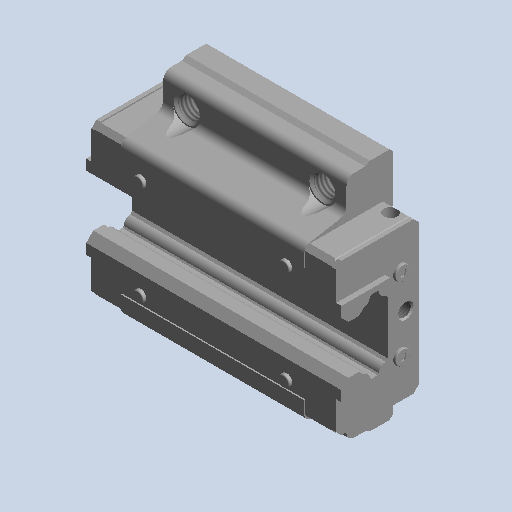
# Autodesk Inventor part: HSR30ASSB-M6F1 Slider-1
Saved by Autodesk Inventor 2022 (Build 260153000, 153)
## iProperties
Part Number: HSR30ASSB-M6F1 Slider-1
Material: Generic
Catalog Web Link: www.cadenas.de
Description: Flange Type - Heavy Load HSR-A Slider-Slider
Vendor: THK
Document SubType Name: Modeling
Designer: partserver
Manufacturer: THK
Mass: 181.354 g
Surface Area: 319.293 cm^2
Volume: 181.354 cm^3
Density: 1 g/cm^3
Appearance: PSOLRGB-192-192-192
Category: PARTsolutions
Company: THK
PSOL_IDENT_0: {$CADENAS_DATA\23d-libs\thk\linear_motion_systems\lm_guide\lm_guide\lm_guide_hsr\four_taped_hole_typ
PSOL_IDENT_1: e\hsr_a\hsr_a_slider.prj},234 {VTYP=3D},{NB=HSR30ASSB-M6F1 Slider-1},{LINA=HSR30ASSB-M6F1 Slider-1},
PSOL_IDENT_2: {NN=Flange Type - Heavy Load HSR-A Slider},{DATE=08.06.2021 00:57:44},{GEOMDATE=03.12.2020 11:07:00}
PSOL_IDENT_3: ,{VERSION=},{LINEID=70},{WBVAR=SO,QZ,GPJ,TH,XY},{WBNUMERIC=XY}  {NB=HSR30ASSB-M6F1 Slider-1},{LINA=H
PSOL_IDENT_4: SR30ASSB-M6F1 Slider-1},{KT=DUMMY},{MN=HSR30A},{SO=SS},{QZ=},{GPJ=B-M6F},{TH=1},{SO1='SS','SS- With
PSOL_IDENT_5: end, side seals','','Without Seals','UU','UU- With end seals (on both ends)','DD','DD- With double,
PSOL_IDENT_6: side, inner seals','ZZ','ZZ- With end, side, inner seals and metal scrapers','KK','KK- With double,
PSOL_IDENT_7: side, inner seals and metal scrapers','SSHH','SSHH- With end, side, inner seals and LaCS','DDHH','DD
PSOL_IDENT_8: HH- With double, side, inner seals and LaCS','ZZHH','ZZHH- With end, side, inner seals and metal scr
PSOL_IDENT_9: apers and LaCS','KKHH','KKHH- With double, side, inner seals and metal scrapers and LaCS'},{M=42.00}
PSOL_IDENT_10: ,{W=90.00},{L=98.00},{B=72.00},{C=52.00},{S=10.00},{L1=70.40},{SST=0.000},{T=9.000},{T1=18.000},{K=3
PSOL_IDENT_11: 5.00},{N=7.00},{H3=7.000},{W1=28.000},{M1=26.000},{LX=98},{LL1=0.000},{SH=58.00},{Z1=2.000},{Z2=2.00
PSOL_IDENT_12: 0},{GPJ1=<'B-M6F','B-M6F'>,'', 'None', 'A-M6F','A-M6F','C-M6F','C-M6F', 'LF-A','LF-A','LF-B','LF-B',
PSOL_IDENT_13: 'SF-A','SF-A','SF-B','SF-B'},{L4=0.95},{ND=4.000},{SE=58.000},{SE3=2.000},{SE4=2.000},{V=38.000},{V
PSOL_IDENT_14: 1=56.000},{V2=4.370},{V3=1.283},{ST=31.717},{SE1=31.717},{SU=1.283},{SE2=1.283},{STT=2.000},{SEE1=2.
PSOL_IDENT_15: 000},{UP=1.283},{QZX='','No','QZ','Yes'},{LP=2},{L3=10.300},{L5=2},{S2=5.500},{L7=0.000},{XX=28.000}
PSOL_IDENT_16: ,{R=2.850},{YY=26.000},{SS=2.500},{ZZ=0.000},{GPJX=2},{X=2},{E0=5.200},{F0=6.200},{D0=5.200},{D2=6.2
PSOL_IDENT_17: 00},{E1=5.200},{SD2=1.00},{XY=1},{WX=11.000},{H1=1.000},{H2=0.400},{RX=19.500},{D=6.200},{LL=5.120},
PSOL_IDENT_18: {TX=1.000},{NOTE=MIN}
NB: HSR30ASSB-M6F1 Slider-1
NN: Flange Type - Heavy Load HSR-A Slider
NT: Slider
NBSYN: $MN.$SO.$QZ.$GPJ.$TH. Slider-$XY.
LINA: HSR30ASSB-M6F1 Slider-1
CATALOG: THK
MN: HSR30A
SO: SS- With end, side seals
QZ: No
GPJ: B-M6F
TH: on
M: 42
W: 90
L: 98
B: 72
C: 52
S: 10
L1: 70.4
SST: 0
T: 9
T1: 18
K: 35
N: 7
H3: 7
W1: 28
M1: 26
LL1: 0
SH: 58
Z1: 2
Z2: 2
ND: 4
SE: 58
SE3: 2
SE4: 2
V: 38
V1: 56
V2: 4.37
V3: 1.283
SU: 1.283
SE2: 1.283
STT: 2
SEE1: 2
L3: 10.3
S2: 5.5
L7: 0
XX: 28
R: 2.85
YY: 26
SS: 2.5
ZZ: 0
E0: 5.2
F0: 6.2
D0: 5.2
D2: 6.2
E1: 5.2
SD2: 1
XY: 1
WX: 11
H1: 1
H2: 0.4
RX: 19.5
D: 6.2
LL: 5.12
TX: 1
NOTE: 0
SUPPLIER: THK
ARTICLENO: HSR30ASSB-M6F1 Slider-1
BOMINFO: HSR30ASSB-M6F1 Slider-1
CREATOR: CADENAS GmbH
Title: HSR30ASSB-M6F1 Slider-1
Author: Cadenas PARTsolutions
Comments: Slider
Autodesk Inventor part; units mm, degrees
sketch "Sketch_17" plane through (0, 0, 0) normal (1, 0, 0) x (0, 1, 0)
  line L0 (33.6, 45) -> (26, 45)
  line L1 (26, 45) -> (24.268, 44)
  line L2 (24.268, 44) -> (20, 44)
  arc A0 (20, 44) -> (17, 41) centre (20, 41) ccw
  line L3 (17, 41) -> (17, 34.3433)
  arc A1 (14.514, 31.3877) -> (17, 34.3433) centre (14, 34.3433) ccw
  line L4 (14.514, 31.3877) -> (3.269, 29.4323)
  arc A2 (3.269, 29.4323) -> (0.783, 26.4767) centre (3.783, 26.4767) ccw
  line L5 (0.783, 26.4767) -> (0.783, 22)
  line L6 (0.783, 22) -> (1.283, 22)
  line L7 (1.283, 22) -> (1.283, -22)
  line L8 (1.283, -22) -> (0.783, -22)
  line L9 (0.783, -22) -> (0.783, -26.4767)
  arc A3 (0.783, -26.4767) -> (3.269, -29.4323) centre (3.783, -26.4767) ccw
  line L10 (3.269, -29.4323) -> (14.514, -31.3877)
  arc A4 (17, -34.3433) -> (14.514, -31.3877) centre (14, -34.3433) ccw
  line L11 (17, -34.3433) -> (17, -41)
  arc A5 (17, -41) -> (20, -44) centre (20, -41) ccw
  line L12 (20, -44) -> (24.268, -44)
  line L13 (24.268, -44) -> (26, -45)
  line L14 (26, -45) -> (33.6, -45)
  line L15 (33.6, -45) -> (35, -43.6)
  line L16 (35, -43.6) -> (35, -25.8)
  line L17 (35, -25.8) -> (34.2, -25)
  line L18 (34.2, -25) -> (34.2, -11)
  line L19 (34.2, -11) -> (35, -10.2)
  line L20 (35, -10.2) -> (35, 10.2)
  line L21 (35, 10.2) -> (34.2, 11)
  line L22 (34.2, 11) -> (34.2, 25)
  line L23 (34.2, 25) -> (35, 25.8)
  line L24 (35, 25.8) -> (35, 43.6)
  line L25 (35, 43.6) -> (33.6, 45)
  constraints: 52 end point, 12 point on circle, 6 centre point
extrude "Extrusion1" add sketch "Sketch_17" along normal mid plane 70.4
sketch "Sketch_28" plane through (0, 0, 36) normal (0, 0, 1) x (1, 0, 0)
  line L0 (-26, 35) -> (-26, 17)
  line L1 (-26, 17) -> (-31, 17)
  line L2 (-31, 17) -> (-30.188, 17.812)
  line L3 (-30.188, 17.812) -> (-30.188, 34.188)
  line L4 (-30.188, 34.188) -> (-31, 35)
  line L5 (-31, 35) -> (-26, 35)
  line L6 (-26, 35) -> (-26, 17)
  constraints: 14 end point
revolve "Revolution1" cut sketch "Sketch_28" angle 360 about axis through (-26, 35, 36) along (0, 1, 0)
thread "Thread1" size "M10x1.5" class "6H" standard "ISO Metric profile" full length
pattern_linear "Rectangular Pattern1" count 2 spacing 52 along (1, 0, 0) count 2 spacing 72 along (0, 0, -1) of "Revolution1"
sketch "Sketch_60" plane through (0, 17, 0) normal (0, 1, 0) x (1, 0, 0)
  line L0 (-31.5, -36) -> (-31.5, -53.5)
  line L1 (-31.5, -53.5) -> (-20.5, -53.5)
  line L2 (-20.5, -53.5) -> (-20.5, -36)
  arc A0 (-20.5, -36) -> (-31.5, -36) centre (-26, -36) ccw
  constraints: 6 end point, 2 point on circle, 1 centre point
extrude "Extrusion2" cut sketch "Sketch_60" against normal blind 35
sketch "Sketch_61" plane through (0, 17, 0) normal (0, 1, 0) x (1, 0, 0)
  arc A0 (-31.5, 36) -> (-20.5, 36) centre (-26, 36) ccw
  line L0 (-20.5, 36) -> (-20.5, 53.5)
  line L1 (-20.5, 53.5) -> (-31.5, 53.5)
  line L2 (-31.5, 53.5) -> (-31.5, 36)
  constraints: 6 end point, 2 point on circle, 1 centre point
extrude "Extrusion3" cut sketch "Sketch_61" against normal blind 17
sketch "Sketch_62" plane through (0, 17, 0) normal (0, 1, 0) x (1, 0, 0)
  line L0 (20.5, -36) -> (20.5, -53.5)
  line L1 (20.5, -53.5) -> (31.5, -53.5)
  line L2 (31.5, -53.5) -> (31.5, -36)
  arc A0 (31.5, -36) -> (20.5, -36) centre (26, -36) ccw
  constraints: 6 end point, 2 point on circle, 1 centre point
extrude "Extrusion4" cut sketch "Sketch_62" against normal blind 17
sketch "Sketch_63" plane through (0, 17, 0) normal (0, 1, 0) x (1, 0, 0)
  arc A0 (20.5, 36) -> (31.5, 36) centre (26, 36) ccw
  line L0 (31.5, 36) -> (31.5, 53.5)
  line L1 (31.5, 53.5) -> (20.5, 53.5)
  line L2 (20.5, 53.5) -> (20.5, 36)
  constraints: 6 end point, 2 point on circle, 1 centre point
extrude "Extrusion5" cut sketch "Sketch_63" against normal blind 17
sketch "Sketch_7" plane through (-45.5, 0, 0) normal (1, 0, 0) x (0, 0, -1)
  line L0 (-29, 2.983) -> (-27.3, 1.283)
  line L1 (-27.3, 1.283) -> (27.3, 1.283)
  line L2 (27.3, 1.283) -> (29, 2.983)
  line L3 (29, 2.983) -> (29, 31)
  line L4 (29, 31) -> (27, 33)
  line L5 (27, 33) -> (-27, 33)
  line L6 (-27, 33) -> (-29, 31)
  line L7 (-29, 31) -> (-29, 2.983)
  constraints: 16 end point
extrude "Extrusion6" add sketch "Sketch_7" along normal blind 10.3
sketch "Sketch_2" plane through (-45.5, 0, 0) normal (1, 0, 0) x (0, 0, -1)
  line L0 (-29, 3.283) -> (-27, 1.283)
  line L1 (-27, 1.283) -> (27, 1.283)
  line L2 (27, 1.283) -> (29, 3.283)
  line L3 (29, 3.283) -> (29, 31)
  line L4 (29, 31) -> (27, 33)
  line L5 (27, 33) -> (-27, 33)
  line L6 (-27, 33) -> (-29, 31)
  line L7 (-29, 31) -> (-29, 3.283)
  constraints: 16 end point
extrude "Extrusion7" add sketch "Sketch_2" against normal blind 3.5
sketch "Sketch_8" plane through (45.5, 0, 0) normal (1, 0, 0) x (0, 0, -1)
  line L0 (-29, 2.983) -> (-27.3, 1.283)
  line L1 (-27.3, 1.283) -> (27.3, 1.283)
  line L2 (27.3, 1.283) -> (29, 2.983)
  line L3 (29, 2.983) -> (29, 31)
  line L4 (29, 31) -> (27, 33)
  line L5 (27, 33) -> (-27, 33)
  line L6 (-27, 33) -> (-29, 31)
  line L7 (-29, 31) -> (-29, 2.983)
  constraints: 16 end point
extrude "Extrusion8" add sketch "Sketch_8" against normal blind 10.3
sketch "Sketch_107" plane through (-35.2, 0, 0) normal (1, 0, 0) x (0, 0, -1)
  line L0 (-10.3, 32.5) -> (10.3, 32.5)
  line L1 (10.3, 32.5) -> (10.3, 34)
  arc A0 (5.5, 34.6) -> (10.3, 34) centre (10.3, 53.5) ccw
  line L2 (5.5, 34.6) -> (-5.5, 34.6)
  arc A1 (-10.3, 34) -> (-5.5, 34.6) centre (-10.3, 53.5) ccw
  line L3 (-10.3, 34) -> (-10.3, 32.5)
  constraints: 8 end point, 4 point on circle, 2 centre point
extrude "Extrusion9" add sketch "Sketch_107" against normal blind 9.8
sketch "Sketch_9" plane through (45.5, 0, 0) normal (1, 0, 0) x (0, 0, -1)
  line L0 (-29, 3.283) -> (-27, 1.283)
  line L1 (-27, 1.283) -> (27, 1.283)
  line L2 (27, 1.283) -> (29, 3.283)
  line L3 (29, 3.283) -> (29, 31)
  line L4 (29, 31) -> (27, 33)
  line L5 (27, 33) -> (-27, 33)
  line L6 (-27, 33) -> (-29, 31)
  line L7 (-29, 31) -> (-29, 3.283)
  constraints: 16 end point
extrude "Extrusion10" add sketch "Sketch_9" along normal blind 3.5
sketch "Sketch_106" plane through (35.2, 0, 0) normal (1, 0, 0) x (0, 0, -1)
  line L0 (-10.3, 32.5) -> (10.3, 32.5)
  line L1 (10.3, 32.5) -> (10.3, 34)
  arc A0 (5.5, 34.6) -> (10.3, 34) centre (10.3, 53.5) ccw
  line L2 (5.5, 34.6) -> (-5.5, 34.6)
  arc A1 (-10.3, 34) -> (-5.5, 34.6) centre (-10.3, 53.5) ccw
  line L3 (-10.3, 34) -> (-10.3, 32.5)
  constraints: 8 end point, 4 point on circle, 2 centre point
extrude "Extrusion11" add sketch "Sketch_106" along normal blind 9.8
sketch "Sketch13" plane through (-45, 34.6, -5.5) normal (0, 1, 0) x (1, 0, 0)
  point P0 (4.68, -5.5)
hole "Hole1" at (-40.32, 34.6, 0) direction (0, -1, 0) diameter 6.2 depth 1
sketch "Sketch14" plane through (35.2, 34.6, 5.5) normal (0, 1, 0) x (1, 0, 0)
  point P0 (5.12, 5.5)
hole "Hole2" at (40.32, 34.6, 0) direction (0, -1, 0) diameter 6.2 depth 1
sketch "Sketch_1" plane through (49, 0, 0) normal (1, 0, 0) x (0, 0, -1)
  line L0 (-29, 35) -> (-29, 0)
  line L1 (-29, 0) -> (29, 0)
  line L2 (29, 0) -> (29, 35)
  line L3 (29, 35) -> (-29, 35)
  constraints: 8 end point
extrude "Extrusion12" cut sketch "Sketch_1" against normal blind 2
sketch "Sketch_6" plane through (-49, 0, 0) normal (1, 0, 0) x (0, 0, -1)
  line L0 (-29, 35) -> (-29, 0)
  line L1 (-29, 0) -> (29, 0)
  line L2 (29, 0) -> (29, 35)
  line L3 (29, 35) -> (-29, 35)
  constraints: 8 end point
extrude "Extrusion13" cut sketch "Sketch_6" along normal blind 2
sketch "Sketch_20" plane through (-47, 0, 0) normal (1, 0, 0) x (0, 0, -1)
  line L0 (-16, 1.283) -> (16, 1.283)
  line L1 (16, 1.283) -> (16, 20)
  line L2 (16, 20) -> (15, 21)
  line L3 (15, 21) -> (-15, 21)
  line L4 (-15, 21) -> (-16, 20)
  line L5 (-16, 20) -> (-16, 1.283)
  constraints: 12 end point
extrude "Extrusion14" add sketch "Sketch_20" against normal blind 2
sketch "Sketch_21" plane through (47, 0, 0) normal (1, 0, 0) x (0, 0, -1)
  line L0 (-16, 1.283) -> (16, 1.283)
  line L1 (16, 1.283) -> (16, 20)
  line L2 (16, 20) -> (15, 21)
  line L3 (15, 21) -> (-15, 21)
  line L4 (-15, 21) -> (-16, 20)
  line L5 (-16, 20) -> (-16, 1.283)
  constraints: 12 end point
extrude "Extrusion15" add sketch "Sketch_21" along normal blind 2
sketch "Sketch_64" plane through (0, 0, 0) normal (1, 0, 0) x (0, 1, 0)
  line L0 (-5.5, 14) -> (-7, 12.5)
  line L1 (-7, 12.5) -> (-7, 7.75)
  line L2 (-7, 7.75) -> (-6.5, 7.25)
  line L3 (-6.5, 7.25) -> (-6.5, 3.75)
  line L4 (-6.5, 3.75) -> (-7, 3.25)
  line L5 (-7, 3.25) -> (-7, -3.25)
  line L6 (-7, -3.25) -> (-6.5, -3.75)
  line L7 (-6.5, -3.75) -> (-6.5, -7.25)
  line L8 (-6.5, -7.25) -> (-7, -7.75)
  line L9 (-7, -7.75) -> (-7, -12.5)
  line L10 (-7, -12.5) -> (-5.5, -14)
  line L11 (-5.5, -14) -> (-0.7, -14)
  line L12 (-0.7, -14) -> (3.9996, -9.3003)
  line L13 (3.9996, -9.3003) -> (8.0794, -9.3003)
  line L14 (8.0794, -9.3003) -> (9.7787, -10.9996)
  arc A0 (12.31, -13.5309) -> (9.7787, -10.9996) centre (9.4399, -13.8696) ccw
  line L15 (12.31, -13.5309) -> (12.7791, -14)
  line L16 (12.7791, -14) -> (15.215, -14)
  line L17 (15.215, -14) -> (15.6905, -13.5245)
  arc A1 (18.2147, -11.0003) -> (15.6905, -13.5245) centre (18.5598, -13.8696) ccw
  line L18 (18.2147, -11.0003) -> (19, -10.215)
  line L19 (19, -10.215) -> (19, 10.215)
  line L20 (19, 10.215) -> (18.2147, 11.0003)
  arc A2 (15.6905, 13.5245) -> (18.2147, 11.0003) centre (18.5598, 13.8696) ccw
  line L21 (15.6905, 13.5245) -> (15.215, 14)
  line L22 (15.215, 14) -> (12.7791, 14)
  line L23 (12.7791, 14) -> (12.31, 13.5309)
  arc A3 (9.7787, 10.9996) -> (12.31, 13.5309) centre (9.4399, 13.8696) ccw
  line L24 (9.7787, 10.9996) -> (8.0794, 9.3003)
  line L25 (8.0794, 9.3003) -> (3.9996, 9.3003)
  line L26 (3.9996, 9.3003) -> (-0.7, 14)
  line L27 (-0.7, 14) -> (-5.5, 14)
  constraints: 56 end point, 8 point on circle, 4 centre point
extrude "Extrusion16" cut sketch "Sketch_64" along normal mid plane 98
sketch "Sketch_4" plane through (0, 0, -14) normal (0, 0, 1) x (1, 0, 0)
  line L0 (47.95, 26) -> (47, 26)
  line L1 (47, 26) -> (47, 28.85)
  line L2 (47, 28.85) -> (47.7125, 28.85)
  arc A0 (47.95, 28.6125) -> (47.7125, 28.85) centre (47.7125, 28.6125) ccw
  line L3 (47.95, 28.6125) -> (47.95, 26)
  line L4 (47.95, 26) -> (47, 26)
  constraints: 10 end point, 2 point on circle, 1 centre point
revolve "Revolution2" add sketch "Sketch_4" angle 360 about axis through (47.95, 26, -14) along (1, 0, 0)
sketch "Sketch_14" plane through (0, 0, -14) normal (0, 0, 1) x (1, 0, 0)
  line L0 (-47, 26) -> (-47.95, 26)
  line L1 (-47.95, 26) -> (-47.95, 28.6125)
  arc A0 (-47.7125, 28.85) -> (-47.95, 28.6125) centre (-47.7125, 28.6125) ccw
  line L2 (-47.7125, 28.85) -> (-47, 28.85)
  line L3 (-47, 28.85) -> (-47, 26)
  line L4 (-47, 26) -> (-47.95, 26)
  constraints: 10 end point, 2 point on circle, 1 centre point
revolve "Revolution3" add sketch "Sketch_14" angle 360 about axis through (-47, 26, -14) along (1, 0, 0)
sketch "Sketch_15" plane through (0, 0, 14) normal (0, 0, 1) x (1, 0, 0)
  line L0 (47.95, 26) -> (47, 26)
  line L1 (47, 26) -> (47, 28.85)
  line L2 (47, 28.85) -> (47.7125, 28.85)
  arc A0 (47.95, 28.6125) -> (47.7125, 28.85) centre (47.7125, 28.6125) ccw
  line L3 (47.95, 28.6125) -> (47.95, 26)
  line L4 (47.95, 26) -> (47, 26)
  constraints: 10 end point, 2 point on circle, 1 centre point
revolve "Revolution4" add sketch "Sketch_15" angle 360 about axis through (47.95, 26, 14) along (1, 0, 0)
sketch "Sketch_16" plane through (0, 0, 14) normal (0, 0, 1) x (1, 0, 0)
  line L0 (-47, 26) -> (-47.95, 26)
  line L1 (-47.95, 26) -> (-47.95, 28.6125)
  arc A0 (-47.7125, 28.85) -> (-47.95, 28.6125) centre (-47.7125, 28.6125) ccw
  line L2 (-47.7125, 28.85) -> (-47, 28.85)
  line L3 (-47, 28.85) -> (-47, 26)
  line L4 (-47, 26) -> (-47.95, 26)
  constraints: 10 end point, 2 point on circle, 1 centre point
revolve "Revolution5" add sketch "Sketch_16" angle 360 about axis through (-47, 26, 14) along (1, 0, 0)
sketch "Sketch_24" plane through (47.95, 0, 0) normal (1, 0, 0) x (0, 0, -1)
  line L0 (12.75, 25.2783) -> (14, 24.5566)
  line L1 (14, 24.5566) -> (15.25, 25.2783)
  line L2 (15.25, 25.2783) -> (15.25, 26.7217)
  line L3 (15.25, 26.7217) -> (14, 27.4434)
  line L4 (14, 27.4434) -> (12.75, 26.7217)
  line L5 (12.75, 26.7217) -> (12.75, 25.2783)
  constraints: 12 end point
extrude "Extrusion17" cut sketch "Sketch_24" against normal blind 0.475
sketch "Sketch_25" plane through (47.95, 0, 0) normal (1, 0, 0) x (0, 0, -1)
  line L0 (-15.25, 25.2783) -> (-14, 24.5566)
  line L1 (-14, 24.5566) -> (-12.75, 25.2783)
  line L2 (-12.75, 25.2783) -> (-12.75, 26.7217)
  line L3 (-12.75, 26.7217) -> (-14, 27.4434)
  line L4 (-14, 27.4434) -> (-15.25, 26.7217)
  line L5 (-15.25, 26.7217) -> (-15.25, 25.2783)
  constraints: 12 end point
extrude "Extrusion18" cut sketch "Sketch_25" against normal blind 0.475
sketch "Sketch_26" plane through (-47.95, 0, 0) normal (1, 0, 0) x (0, 0, -1)
  line L0 (12.75, 25.2783) -> (14, 24.5566)
  line L1 (14, 24.5566) -> (15.25, 25.2783)
  line L2 (15.25, 25.2783) -> (15.25, 26.7217)
  line L3 (15.25, 26.7217) -> (14, 27.4434)
  line L4 (14, 27.4434) -> (12.75, 26.7217)
  line L5 (12.75, 26.7217) -> (12.75, 25.2783)
  constraints: 12 end point
extrude "Extrusion19" cut sketch "Sketch_26" along normal blind 0.475
sketch "Sketch_27" plane through (-47.95, 0, 0) normal (1, 0, 0) x (0, 0, -1)
  line L0 (-15.25, 25.2783) -> (-14, 24.5566)
  line L1 (-14, 24.5566) -> (-12.75, 25.2783)
  line L2 (-12.75, 25.2783) -> (-12.75, 26.7217)
  line L3 (-12.75, 26.7217) -> (-14, 27.4434)
  line L4 (-14, 27.4434) -> (-15.25, 26.7217)
  line L5 (-15.25, 26.7217) -> (-15.25, 25.2783)
  constraints: 12 end point
extrude "Extrusion20" cut sketch "Sketch_27" along normal blind 0.475
sketch "Sketch_12" plane through (0, 0, 0) normal (0, 0, 1) x (1, 0, 0)
  line L0 (-45.5, 32.5) -> (-45, 33)
  line L1 (-45, 33) -> (-45.5, 33)
  line L2 (-45.5, 33) -> (-45.5, 32.5)
  constraints: 6 end point
extrude "Extrusion21" cut sketch "Sketch_12" along normal mid plane 58
sketch "Sketch_13" plane through (0, 0, 0) normal (0, 0, 1) x (1, 0, 0)
  line L0 (45, 33) -> (45.5, 32.5)
  line L1 (45.5, 32.5) -> (45.5, 33)
  line L2 (45.5, 33) -> (45, 33)
  constraints: 6 end point
extrude "Extrusion22" cut sketch "Sketch_13" along normal mid plane 58
sketch "Sketch_90" plane through (0, 0, 0) normal (0, 1, 0) x (-1, 0, 0)
  line L0 (-45, -29) -> (-45.5, -28.5)
  line L1 (-45.5, -28.5) -> (-45.5, -29)
  line L2 (-45.5, -29) -> (-45, -29)
  constraints: 6 end point
extrude "Extrusion23" cut sketch "Sketch_90" along normal blind 35
sketch "Sketch_91" plane through (0, 0, 0) normal (0, 1, 0) x (-1, 0, 0)
  line L0 (45.5, -28.5) -> (45, -29)
  line L1 (45, -29) -> (45.5, -29)
  line L2 (45.5, -29) -> (45.5, -28.5)
  constraints: 6 end point
extrude "Extrusion24" cut sketch "Sketch_91" along normal blind 35
sketch "Sketch_92" plane through (0, 0, 0) normal (0, 1, 0) x (-1, 0, 0)
  line L0 (-45, 29) -> (-45.5, 29)
  line L1 (-45.5, 29) -> (-45.5, 28.5)
  line L2 (-45.5, 28.5) -> (-45, 29)
  constraints: 6 end point
extrude "Extrusion25" cut sketch "Sketch_92" along normal blind 35
sketch "Sketch_93" plane through (0, 0, 0) normal (0, 1, 0) x (-1, 0, 0)
  line L0 (45.5, 28.5) -> (45.5, 29)
  line L1 (45.5, 29) -> (45, 29)
  line L2 (45, 29) -> (45.5, 28.5)
  constraints: 6 end point
extrude "Extrusion26" cut sketch "Sketch_93" along normal blind 35
sketch "Sketch34" plane through (47, 0, 0) normal (1, 0, 0) x (0, 0, -1)
  point P0 (0, 28)
hole "Hole3" at (47, 28, 0) direction (-1, 0, 0) diameter 4.917 depth 6 tip angle 120 countersink diameter 6 countersink angle 90 thread size "M6x1" class "6H" standard "ISO Metric profile"
sketch "Sketch35" plane through (-47, 0, 0) normal (-1, 0, 0) x (0, 0, 1)
  point P0 (0, 28)
hole "Hole4" at (-47, 28, 0) direction (1, 0, 0) diameter 4.917 depth 6 tip angle 120 countersink diameter 6 countersink angle 90 thread size "M6x1" class "6H" standard "ISO Metric profile"
sketch "Sketch_34" plane through (0, 0, -19) normal (0, 0, 1) x (1, 0, 0)
  line L0 (-28, 4.37) -> (-28, 0)
  line L1 (-28, 0) -> (-29.748, 0)
  arc A0 (-30.185, 0.437) -> (-29.748, 0) centre (-29.748, 0.437) ccw
  line L2 (-30.185, 0.437) -> (-30.185, 4.37)
  line L3 (-30.185, 4.37) -> (-28, 4.37)
  line L4 (-28, 4.37) -> (-28, 0)
  constraints: 10 end point, 2 point on circle, 1 centre point
revolve "Revolution6" add sketch "Sketch_34" angle 360 about axis through (-28, 4.37, -19) along (0, 1, 0)
sketch "Sketch_35" plane through (0, 0, -19) normal (0, 0, 1) x (1, 0, 0)
  line L0 (28, 4.37) -> (28, 0)
  line L1 (28, 0) -> (26.252, 0)
  arc A0 (25.815, 0.437) -> (26.252, 0) centre (26.252, 0.437) ccw
  line L2 (25.815, 0.437) -> (25.815, 4.37)
  line L3 (25.815, 4.37) -> (28, 4.37)
  line L4 (28, 4.37) -> (28, 0)
  constraints: 10 end point, 2 point on circle, 1 centre point
revolve "Revolution7" add sketch "Sketch_35" angle 360 about axis through (28, 4.37, -19) along (0, 1, 0)
sketch "Sketch_37" plane through (0, 0, 19) normal (0, 0, 1) x (1, 0, 0)
  line L0 (-28, 4.37) -> (-28, 0)
  line L1 (-28, 0) -> (-29.748, 0)
  arc A0 (-30.185, 0.437) -> (-29.748, 0) centre (-29.748, 0.437) ccw
  line L2 (-30.185, 0.437) -> (-30.185, 4.37)
  line L3 (-30.185, 4.37) -> (-28, 4.37)
  line L4 (-28, 4.37) -> (-28, 0)
  constraints: 10 end point, 2 point on circle, 1 centre point
revolve "Revolution8" add sketch "Sketch_37" angle 360 about axis through (-28, 4.37, 19) along (0, 1, 0)
sketch "Sketch_38" plane through (0, 0, 19) normal (0, 0, 1) x (1, 0, 0)
  line L0 (28, 4.37) -> (28, 0)
  line L1 (28, 0) -> (26.252, 0)
  arc A0 (25.815, 0.437) -> (26.252, 0) centre (26.252, 0.437) ccw
  line L2 (25.815, 0.437) -> (25.815, 4.37)
  line L3 (25.815, 4.37) -> (28, 4.37)
  line L4 (28, 4.37) -> (28, 0)
  constraints: 10 end point, 2 point on circle, 1 centre point
revolve "Revolution9" add sketch "Sketch_38" angle 360 about axis through (28, 4.37, 19) along (0, 1, 0)
sketch "Sketch_98" plane through (40.4, 0, 0) normal (1, 0, 0) x (0, 0, -1)
  line L0 (-23.8, 28.8) -> (-29, 28.8)
  line L1 (-29, 28.8) -> (-29, 31.4)
  line L2 (-29, 31.4) -> (-23.8, 31.4)
  line L3 (-23.8, 31.4) -> (-23.8, 28.8)
  line L4 (-23.8, 28.8) -> (-29, 28.8)
  constraints: 10 end point
revolve "Revolution10" cut sketch "Sketch_98" angle 360 about axis through (40.4, 28.8, 23.8) along (0, 0, -1)
sketch "Sketch41" plane through (35.2, 2.983, -29) normal (0, 0, -1) x (-1, 0, 0)
  point P0 (-5.2, 25.817)
hole "Hole5" at (40.4, 28.8, -29) direction (0, 0, 1) diameter 5.2 depth 5.2
sketch "Sketch_100" plane through (-40.4, 0, 0) normal (1, 0, 0) x (0, 0, -1)
  line L0 (-23.8, 28.8) -> (-29, 28.8)
  line L1 (-29, 28.8) -> (-29, 31.4)
  line L2 (-29, 31.4) -> (-23.8, 31.4)
  line L3 (-23.8, 31.4) -> (-23.8, 28.8)
  line L4 (-23.8, 28.8) -> (-29, 28.8)
  constraints: 10 end point
revolve "Revolution11" cut sketch "Sketch_100" angle 360 about axis through (-40.4, 28.8, 23.8) along (0, 0, -1)
sketch "Sketch43" plane through (-35.2, 2.983, -29) normal (0, 0, -1) x (-1, 0, 0)
  point P0 (5.2, 25.817)
hole "Hole6" at (-40.4, 28.8, -29) direction (0, 0, 1) diameter 5.2 depth 5.2
ref_plane "4TRACK_XY" through (0, 0, 0) normal (1, 0, 0) x (0, 0, -1)
ref_plane "4TRACK_YZ" through (0, 0, 0) normal (0, 0, -1) x (0, 1, 0)
ref_plane "4TRACK_ZX" through (0, 0, 0) normal (0, 1, 0) x (1, 0, 0)
ref_plane "niple_XY" through (-47, 28, 0) normal (1, 0, 0) x (0, 0, -1)
ref_plane "niple_YZ" through (-47, 28, 0) normal (0, 0, -1) x (0, 1, 0)
ref_plane "niple_ZX" through (-47, 28, 0) normal (0, 1, 0) x (1, 0, 0)
ref_plane "niple2_XY" through (47, 28, 0) normal (1, 0, 0) x (0, 0, -1)
ref_plane "niple2_YZ" through (47, 28, 0) normal (0, 0, -1) x (0, 1, 0)
ref_plane "niple2_ZX" through (47, 28, 0) normal (0, 1, 0) x (1, 0, 0)
body "Solid1"
